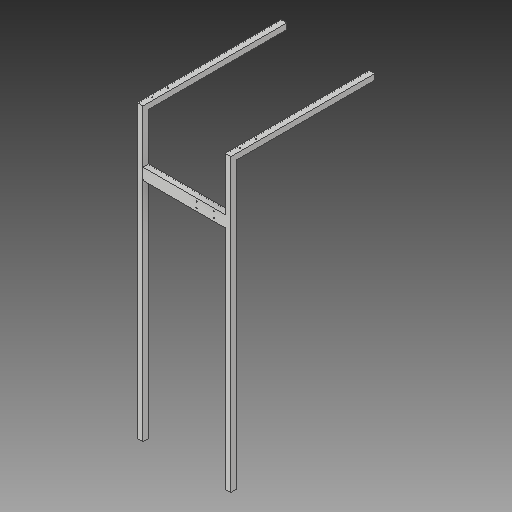
# Autodesk Inventor part: armFrame
Saved by Autodesk Inventor 2019 (Build 230136000, 136)
## iProperties
Created: 2018-02-07
Part Number: armFrame
Material: Generic
Document SubType Name: Modeling
Designer: steele
Density: 1 g/cm^3
Appearance: Default
Author: steele
Autodesk Inventor part; units mm, degrees
ref_plane "YZ Plane" through (0, 0, 0) normal (1, 0, 0) x (0, 1, 0)
ref_plane "XZ Plane" through (0, 0, 0) normal (0, 1, 0) x (-1, 0, 0)
ref_plane "XY Plane" through (0, 0, 0) normal (0, 0, 1) x (1, 0, 0)
sketch "Sketch1" plane through (0, 0, 0) normal (0, 1, 0) x (-1, 0, 0)
  line L0 (12.7, 12.7) -> (-12.7, 12.7)
  line L1 (-12.7, 12.7) -> (-12.7, -12.7)
  line L2 (-12.7, -12.7) -> (12.7, -12.7)
  line L3 (12.7, -12.7) -> (12.7, 12.7)
  line L4 (12.7, 12.7) -> (-12.7, -12.7) construction
  line L5 (-12.7, 12.7) -> (12.7, -12.7) construction
  line L6 (9.525, 9.525) -> (-9.525, 9.525)
  line L7 (-9.525, 9.525) -> (-9.525, -9.525)
  line L8 (-9.525, -9.525) -> (9.525, -9.525)
  line L9 (9.525, -9.525) -> (9.525, 9.525)
  line L10 (9.525, 9.525) -> (-9.525, -9.525) construction
  line L11 (-9.525, 9.525) -> (9.525, -9.525) construction
  point P0 (0, 0)
  dimension "d0" = 25.4
  dimension "d1" = 3.175
  constraints: 24 end point, 4 midpoint, 4 parallel, 4 perpendicular, 2 horizontal
  measures "d0" distance of L0.start L0.end
  measures "d1" distance between parallel lines of L0 L6
sketch3d "3D Sketch2"
  line L0 (0, 0, 0) -> (0, 1270, 0)
  line L1 (0, 1270, 0) -> (0, 1270, -838.2)
  line L2 (0, 1270, -838.2) -> (-387.35, 1270, -838.2)
  line L3 (-387.35, 1270, -838.2) -> (-387.35, 1270, 0)
  line L4 (-387.35, 1270, 0) -> (-387.35, 0, 0)
  dimension "d4" = 1270
  dimension "d5" = 387.35
  dimension "d6" = 1270
  dimension "d7" = 838.2
sweep "Sweep1" add profiles "Sketch1" path "3D Sketch2"
sketch "Sketch5" plane through (-374.65, 0, 12.7) normal (1, 0, 0) x (0, 0, -1)
  line L0 (0, 1282.7) -> (0, 0) projected
  line L1 (25.4, 1257.3) -> (25.4, 0) projected
  line L2 (0, 998.1547) -> (25.4, 998.1547)
  line L3 (25.4, 998.1547) -> (25.4, 1048.9547)
  line L4 (25.4, 1048.9547) -> (0, 1048.9547)
  line L5 (0, 1048.9547) -> (0, 998.1547)
  line L6 (3.175, 1001.3297) -> (22.225, 1001.3297)
  line L7 (22.225, 1001.3297) -> (22.225, 1045.7797)
  line L8 (22.225, 1045.7797) -> (3.175, 1045.7797)
  line L9 (3.175, 1045.7797) -> (3.175, 1001.3297)
  line L10 (3.175, 1001.3297) -> (22.225, 1045.7797) construction
  line L11 (22.225, 1001.3297) -> (3.175, 1045.7797) construction
  point P0 (12.7, 0)
  point P1 (12.7, 1023.5547)
  dimension "d26" = 50.8
  dimension "d27" = 3.175
  dimension "d28" = 3.175
  dimension "d29" = 3.175
  dimension "d30" = 3.175
  dimension "d33" = 233.7453
  constraints: 20 end point, 4 parallel, 2 horizontal, 2 midpoint, 2 perpendicular, 2 point on line
  measures "d26" distance of L3.end L2.end
  measures "d27" distance between parallel lines of L6 L2
  measures "d28" distance between parallel lines of L8 L4
  measures "d29" distance between parallel lines of L0 L9
  measures "d30" distance between parallel lines of L1 L7
  measures "d33" distance from line of L4 L0.start
extrude "Extrusion1" add sketch "Sketch5" along normal blind 361.95
sketch "Sketch6" plane through (-400.05, 1282.7, -850.9) normal (0, 1, 0) x (1, 0, 0)
  line L0 (412.75, 0) -> (0, 0) projected
  line L1 (25.4, -25.4) -> (387.477, -25.4)
  line L2 (387.477, -25.4) -> (387.477, 0)
  line L3 (387.477, 0) -> (25.4, 0)
  line L4 (25.4, 0) -> (25.4, -25.4)
  point P0 (400.05, -850.9)
  dimension "d36" = 362.077
  constraints: 8 end point, 2 parallel, 1 horizontal, 1 perpendicular, 1 point on line
  measures "d36" distance of L1.start L1.end
extrude "Extrusion2" cut sketch "Sketch6" against normal through all
sketch "Sketch7" plane through (-12.7, 1282.7, 12.7) normal (0, 1, 0) x (1, 0, 0)
  point P0 (12.7, 53.975)
hole "Hole4" at (0, 1282.7, -41.275) direction (0, -1, 0) diameter 5.1054 depth 3.175
sketch "Sketch8" plane through (-12.7, 1257.3, -12.7) normal (0, -1, 0) x (1, 0, 0)
  point P0 (12.7, -28.575)
hole "Hole6" at (0, 1257.3, -41.275) direction (0, 1, 0) diameter 5.1054 depth 3.175
sketch "Sketch9" plane through (-12.7, 1282.7, 12.7) normal (0, 1, 0) x (1, 0, 0)
  point P0 (12.7, 123.825)
hole "Hole8" at (0, 1282.7, -111.125) direction (0, -1, 0) diameter 5.08 depth 3.175
sketch "Sketch10" plane through (-12.7, 1257.3, -12.7) normal (0, -1, 0) x (1, 0, 0)
  point P0 (12.7, -98.425)
hole "Hole10" at (0, 1257.3, -111.125) direction (0, 1, 0) diameter 5.08 depth 3.175
sketch "Sketch11" plane through (-400.05, 1282.7, -850.9) normal (0, 1, 0) x (1, 0, 0)
  point P0 (12.7, -809.625)
hole "Hole12" at (-387.35, 1282.7, -41.275) direction (0, -1, 0) diameter 5.08 depth 3.175
sketch "Sketch12" plane through (-400.05, 1257.3, -12.7) normal (0, -1, 0) x (1, 0, 0)
  point P0 (12.7, -28.575)
hole "Hole14" at (-387.35, 1257.3, -41.275) direction (0, 1, 0) diameter 5.08 depth 3.175
sketch "Sketch13" plane through (-400.05, 1282.7, -850.9) normal (0, 1, 0) x (1, 0, 0)
  point P0 (12.7, -739.775)
hole "Hole16" at (-387.35, 1282.7, -111.125) direction (0, -1, 0) diameter 5.08 depth 3.175
sketch "Sketch14" plane through (-400.05, 1257.3, -12.7) normal (0, -1, 0) x (1, 0, 0)
  point P0 (12.7, -98.425)
hole "Hole18" at (-387.35, 1257.3, -111.125) direction (0, 1, 0) diameter 5.08 depth 3.175
sketch "Sketch19" plane through (-400.05, 1282.7, -850.9) normal (0, 1, 0) x (1, 0, 0)
  line L0 (412.75, -863.6) -> (412.75, 0) projected
  line L1 (0, 0) -> (412.75, 0)
  line L2 (412.75, 0) -> (412.75, -228.6)
  line L3 (412.75, -228.6) -> (0, -228.6)
  line L4 (0, -228.6) -> (0, 0)
  point P0 (400.05, -850.9)
  dimension "d121" = 228.6
  constraints: 8 end point, 2 parallel, 1 horizontal, 1 perpendicular, 1 point on line
  measures "d121" distance of L1.end L2.end
extrude "Extrusion3" cut sketch "Sketch19" against normal through all
sketch "Sketch20" plane through (-400.05, 0, 12.7) normal (0, 0, 1) x (1, 0, 0)
  line L0 (261.6184, 1010.8547) -> (337.8184, 1010.8547) construction
  line L1 (337.8184, 1010.8547) -> (337.8184, 1036.2547) construction
  line L2 (337.8184, 1036.2547) -> (261.6184, 1036.2547) construction
  line L3 (261.6184, 1036.2547) -> (261.6184, 1010.8547) construction
  line L4 (261.6184, 1010.8547) -> (337.8184, 1036.2547) construction
  line L5 (337.8184, 1010.8547) -> (261.6184, 1036.2547) construction
  line L6 (25.4, 998.1547) -> (387.35, 998.1547) construction
  point P0 (400.05, 0)
  point P1 (299.7184, 1023.5547)
  dimension "d124" = 76.2
  dimension "d125" = 25.4
  dimension "d126" = 25.4
  constraints: 12 end point, 4 coincident, 3 parallel, 2 midpoint, 1 horizontal, 1 perpendicular
  measures "d124" distance of L0.start L0.end
  measures "d125" distance of L1.end L0.end
  measures "d126" distance from line of point (299.718, 1023.555) L6
hole "Hole28" at (-138.4316, 1036.2547, 12.7) at (-62.2316, 1036.2547, 12.7) at (-62.2316, 1010.8547, 12.7) at (-138.4316, 1010.8547, 12.7) direction (0, 0, -1) diameter 5.1054 depth 25.4 tip angle 118
equation "\"d1\" = wallThickness"
equation "\"d4\" = height"
equation "\"d5\" = width"
equation "\"d6\" = height"
equation "\"d7\" = length"
equation "\"d31\" = motorSupportWidth"
equation "\"d36\" = removeExtraBrace"
equation "\"width\" = 387.35"
equation "\"length\" = 838.2"
equation "\"wallThickness\" = 3.175"
equation "\"motorSupportWidth\" = 361.95"
equation "\"removeExtraBrace\" = 362.077"
equation "\"height\" = 1270"
body "Solid1"
